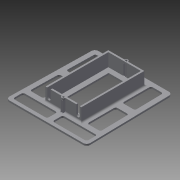
# Autodesk Inventor part: control pod layer b
Saved by Autodesk Inventor 2014 SP1 (Build 180222100, 222)
## iProperties
Created: 2017-06-28
Part Number: control pod layer b
Material: Generic
Document SubType Name: Modeling
Designer: kteo17
Density: 1 g/cm^3
Appearance: Default
Author: kteo17
Autodesk Inventor part; units mm, degrees
ref_plane "YZ Plane" through (0, 0, 0) normal (1, 0, 0) x (0, 1, 0)
ref_plane "XZ Plane" through (0, 0, 0) normal (0, 1, 0) x (-1, 0, 0)
ref_plane "XY Plane" through (0, 0, 0) normal (0, 0, 1) x (1, 0, 0)
sketch "Sketch1" plane through (0, 0, 0) normal (0, 0, 1) x (1, 0, 0)
  line L0 (3.175, 0) -> (146.685, 0)
  line L1 (149.86, 161.925) -> (0, 161.925)
  line L2 (0, 161.925) -> (3.175, 0)
  line L3 (149.86, 161.925) -> (146.685, 0)
  point P0 (0, 0)
  dimension "d74" = 161.925
  dimension "d75" = 143.51
  dimension "d76" = 149.86
  constraints: 8 end point, 1 horizontal, 1 parallel
  measures "d74" distance between parallel lines of L0 L1
  measures "d75" distance of L0.start L0.end
  measures "d76" distance of L1.start L1.end
extrude "Extrusion1" add sketch "Sketch1" along normal blind 3.048
fillet "Fillet1" radius 6.35 3 edges at (149.86, 161.925, 1.524) (146.685, 0, 1.524) (0, 161.925, 1.524)
sketch "Sketch4" plane through (0, 0, 3.048) normal (0, 0, 1) x (1, 0, 0)
  line L0 (44.7675, 16.764) -> (105.0925, 16.764)
  line L1 (105.0925, 16.764) -> (105.0925, 127)
  line L2 (105.0925, 127) -> (44.7675, 127)
  line L3 (44.7675, 127) -> (44.7675, 16.764)
  line L4 (44.7675, 16.764) -> (105.0925, 127) construction
  line L5 (105.0925, 16.764) -> (44.7675, 127) construction
  line L6 (41.5925, 13.589) -> (108.2675, 13.589)
  line L7 (108.2675, 13.589) -> (108.2675, 130.175)
  line L8 (108.2675, 130.175) -> (41.5925, 130.175)
  line L9 (41.5925, 130.175) -> (41.5925, 13.589)
  line L10 (193.675, 0) -> (193.675, 12.7)
  line L11 (3.175, 0) -> (140.4583, 0) projected
  point P0 (0, 0)
  dimension "d12" = 110.236
  dimension "d50" = 3.175
  dimension "d51" = 3.175
  dimension "d52" = 3.175
  dimension "d67" = 3.175
  dimension "d78" = 66.675
  dimension "d126" = 13.589
  constraints: 22 end point, 4 parallel, 2 horizontal, 2 perpendicular
  measures "d12" distance of L1.end L0.end
  measures "d50" distance between parallel lines of L2 L8
  measures "d51" distance between parallel lines of L7 L1
  measures "d52" distance between parallel lines of L0 L6
  measures "d67" distance between parallel lines of L9 L3
  measures "d78" distance of L7.end L8.end
  measures "d126" distance between parallel lines of L11 L6
extrude "Extrusion4" add sketch "Sketch4" along normal blind 24.13
sketch "Sketch5" plane through (0, 0, 27.178) normal (0, 0, 1) x (1, 0, 0)
  line L0 (41.5925, 13.589) -> (108.2675, 13.589) projected
  line L1 (108.2675, 130.175) -> (41.5925, 130.175) projected
  arc A0 (78.105, 130.175) -> (71.755, 130.175) centre (74.93, 130.175) ccw
  arc A1 (71.755, 13.589) -> (78.105, 13.589) centre (74.93, 13.589) ccw
  point P0 (0, 0)
  dimension "d127" = 3.175
  constraints: 4 point on circle, 4 point on line, 2 centre point, 2 midpoint
  measures "d127" radius of A0
extrude "Extrusion5" add sketch "Sketch5" against normal blind 3.175
sketch "Sketch6" plane through (41.5925, 130.175, 3.048) normal (0, 1, 0) x (1, 0, 0)
  line L0 (0, 0) -> (66.675, 0) projected
  line L1 (30.1625, -20.955) -> (36.5125, -20.955)
  line L2 (36.5125, -20.955) -> (36.5125, 0)
  line L3 (36.5125, 0) -> (30.1625, 0)
  line L4 (30.1625, 0) -> (30.1625, -20.955)
  point P0 (-41.5925, 3.048)
  constraints: 8 end point, 2 parallel, 1 horizontal, 1 perpendicular, 1 point on line
extrude "Extrusion6" cut sketch "Sketch6" against normal blind 127
sketch "Sketch9" plane through (0, 0, 27.178) normal (0, 0, 1) x (1, 0, 0)
  arc A0 (71.755, 13.589) -> (78.105, 13.589) centre (74.93, 13.589) ccw projected
  arc A1 (78.105, 130.175) -> (71.755, 130.175) centre (74.93, 130.175) ccw projected
  circle A2 centre (74.93, 130.175) radius 1.5875
  circle A3 centre (74.93, 13.589) radius 1.5875
  point P0 (0, 0)
  constraints: 2 centre point, 2 coincident
extrude "Extrusion9" cut sketch "Sketch9" against normal blind 2.54
sketch "Sketch10" plane through (108.2675, 130.175, 27.178) normal (0, 1, 0) x (1, 0, 0)
  line L0 (0, 0) -> (-30.1625, 0) projected
  line L1 (-3.175, 0) -> (-9.525, 0)
  line L2 (-9.525, 0) -> (-9.525, 15.875)
  line L3 (-6.35, 22.225) -> (-6.35, 22.225)
  line L4 (-3.175, 15.875) -> (-3.175, 0)
  line L5 (-63.5, 0) -> (-57.15, 0)
  line L6 (-57.15, 0) -> (-57.15, 15.875)
  line L7 (-60.325, 22.225) -> (-60.325, 22.225)
  line L8 (-63.5, 15.875) -> (-63.5, 0)
  arc A0 (-57.15, 15.875) -> (-63.5, 15.875) centre (-60.325, 15.875) ccw
  arc A1 (-3.175, 15.875) -> (-9.525, 15.875) centre (-6.35, 15.875) ccw
  point P0 (-108.2675, 27.178)
  constraints: 16 end point, 4 parallel, 4 point on circle, 2 centre point, 2 horizontal, 2 perpendicular, 2 point on line, 2 tangent
extrude "Extrusion10" cut sketch "Sketch10" against normal blind 25.4
fillet "Fillet3" radius 3.175 6 edges at (93.1863, 130.175, 3.048) (56.6738, 130.175, 3.048) (108.2675, 71.882, 3.048) (93.1863, 13.589, 3.048) (56.6738, 13.589, 3.048) (41.5925, 71.882, 3.048)
sketch "Sketch15" plane through (0, 0, 3.048) normal (0, 0, 1) x (1, 0, 0)
  line L0 (72.9998, 133.35) -> (74.0715, 133.35)
  line L1 (74.0715, 133.35) -> (74.0715, 126.111)
  line L2 (74.0715, 126.111) -> (72.9998, 126.111)
  line L3 (72.9998, 126.111) -> (72.9998, 133.35)
  line L4 (76.876, 133.35) -> (75.7704, 133.35)
  line L5 (75.7704, 133.35) -> (75.7704, 126.111)
  line L6 (75.7704, 126.111) -> (76.876, 126.111)
  line L7 (76.876, 126.111) -> (76.876, 133.35)
  line L8 (73.0082, 16.7637) -> (74.08, 16.7637)
  line L9 (74.08, 16.7637) -> (74.08, 10.4137)
  line L10 (74.08, 10.4137) -> (73.0082, 10.4137)
  line L11 (73.0082, 10.4137) -> (73.0082, 16.7637)
  line L12 (76.8845, 10.4137) -> (75.7789, 10.4137)
  line L13 (75.7789, 10.4137) -> (75.7789, 16.7637)
  line L14 (75.7789, 16.7637) -> (76.8845, 16.7637)
  line L15 (76.8845, 16.7637) -> (76.8845, 10.4137)
  point P0 (0, 0)
  constraints: 32 end point, 8 parallel, 4 horizontal, 4 perpendicular
extrude "Extrusion15" add sketch "Sketch15" along normal blind 20.7772
sketch "Sketch16" plane through (75.7704, 133.35, 3.048) normal (0, 1, 0) x (1, 0, 0)
  line L0 (-3.175, 0) -> (1.5875, 0)
  line L1 (1.5875, 0) -> (1.5875, -0.254)
  line L2 (1.5875, -0.254) -> (-3.175, -0.254)
  line L3 (-3.175, -0.254) -> (-3.175, 0)
  point P0 (-75.7704, 3.048)
  dimension "d58" = 0.254
  constraints: 8 end point, 2 parallel, 1 horizontal, 1 perpendicular
  measures "d58" distance of L0.end L1.end
extrude "Extrusion16" cut sketch "Sketch16" against normal blind 127
fillet "Fillet4" radius 6.35 1 edges at (3.175, 0, 1.524)
sketch "Sketch19" plane through (0, 0, 3.048) normal (0, 0, 1) x (1, 0, 0)
  line L0 (54.2925, 25.8383) -> (95.5675, 25.8383)
  line L1 (95.5675, 25.8383) -> (95.5675, 117.9257)
  line L2 (95.5675, 117.9257) -> (54.2925, 117.9257)
  line L3 (54.2925, 117.9257) -> (54.2925, 25.8383)
  line L4 (54.2925, 25.8383) -> (95.5675, 117.9257) construction
  line L5 (95.5675, 25.8383) -> (54.2925, 117.9257) construction
  point P0 (0, 0)
  point P1 (74.93, 71.882)
  constraints: 12 end point, 2 midpoint, 2 parallel, 1 horizontal, 1 perpendicular
extrude "Extrusion18" cut sketch "Sketch19" against normal blind 3.048
sketch "Sketch21" plane through (0, 0, 3.048) normal (0, 0, 1) x (1, 0, 0)
  arc A0 (149.733, 155.4505) -> (143.3843, 161.925) centre (143.3843, 155.575) ccw projected
  line L0 (143.3843, 139.7) -> (143.3843, 152.4)
  line L1 (6.4757, 152.4) -> (6.4757, 139.7)
  line L2 (79.8843, 152.4) -> (79.8843, 139.7)
  line L3 (69.9757, 152.4) -> (69.9757, 139.7)
  line L4 (140.2093, 155.575) -> (83.0593, 155.575)
  line L5 (66.8007, 155.575) -> (9.6507, 155.575)
  line L6 (9.6507, 136.525) -> (66.8007, 136.525)
  line L7 (83.0593, 136.525) -> (140.2093, 136.525)
  arc A1 (9.6507, 155.575) -> (6.4757, 152.4) centre (9.6507, 152.4) ccw
  arc A2 (6.4757, 139.7) -> (9.6507, 136.525) centre (9.6507, 139.7) ccw
  arc A3 (66.8007, 136.525) -> (69.9757, 139.7) centre (66.8007, 139.7) ccw
  arc A4 (69.9757, 152.4) -> (66.8007, 155.575) centre (66.8007, 152.4) ccw
  arc A5 (83.0593, 155.575) -> (79.8843, 152.4) centre (83.0593, 152.4) ccw
  arc A6 (79.8843, 139.7) -> (83.0593, 136.525) centre (83.0593, 139.7) ccw
  arc A7 (140.2093, 136.525) -> (143.3843, 139.7) centre (140.2093, 139.7) ccw
  arc A8 (143.3843, 152.4) -> (140.2093, 155.575) centre (140.2093, 152.4) ccw
  point P0 (0, 0)
  dimension "d97" = 3.175
  dimension "d111" = 19.05
  dimension "d112" = 19.05
  dimension "d113" = 63.5
  dimension "d114" = 63.5
  constraints: 16 end point, 16 point on circle, 16 tangent, 8 centre point, 7 equal radius, 6 perpendicular, 5 parallel, 2 horizontal, 2 point on line
  measures "d97" radius of A1
  measures "d111" distance between parallel lines of L6 L5
  measures "d112" distance between parallel lines of L4 L7
  measures "d113" distance between parallel lines of L3 L1
  measures "d114" distance between parallel lines of L0 L2
extrude "Extrusion20" cut sketch "Sketch21" against normal blind 3.048
sketch "Sketch22" plane through (0, 0, 3.048) normal (0, 0, 1) x (1, 0, 0)
  line L0 (66.8007, 136.525) -> (9.6507, 136.525) projected
  line L1 (146.8071, 6.2255) -> (149.733, 155.4505) projected
  line L2 (0.127, 155.4505) -> (3.0529, 6.2255) projected
  line L3 (31.115, 127) -> (12.6633, 127)
  line L4 (118.745, 127) -> (137.1967, 127)
  line L5 (15.5083, 7.9375) -> (31.75, 7.9375)
  line L6 (118.745, 7.9375) -> (134.9867, 7.9375)
  line L7 (13.5815, 73.8187) -> (31.115, 73.8187)
  line L8 (14.59, 61.1187) -> (31.75, 61.1187)
  line L9 (118.745, 61.1187) -> (135.905, 61.1187)
  line L10 (118.745, 73.8187) -> (136.2785, 73.8187)
  line L11 (9.4889, 123.7628) -> (10.4071, 76.9315)
  line L12 (11.4157, 57.8815) -> (12.3339, 11.0503)
  line L13 (34.29, 123.825) -> (34.29, 76.9937)
  line L14 (34.925, 57.9437) -> (34.925, 11.1125)
  line L15 (115.57, 123.825) -> (115.57, 76.9937)
  line L16 (115.57, 57.9437) -> (115.57, 11.1125)
  line L17 (140.3711, 123.7628) -> (139.4529, 76.9315)
  line L18 (139.0793, 57.8815) -> (138.1611, 11.0503)
  arc A0 (12.6633, 127) -> (9.4889, 123.7628) centre (12.6633, 123.825) ccw
  arc A1 (34.29, 123.825) -> (31.115, 127) centre (31.115, 123.825) ccw
  arc A2 (34.925, 57.9437) -> (31.75, 61.1187) centre (31.75, 57.9437) ccw
  arc A3 (14.59, 61.1187) -> (11.4157, 57.8815) centre (14.59, 57.9437) ccw
  arc A4 (12.3339, 11.0503) -> (15.5083, 7.9375) centre (15.5083, 11.1125) ccw
  arc A5 (31.75, 7.9375) -> (34.925, 11.1125) centre (31.75, 11.1125) ccw
  arc A6 (115.57, 11.1125) -> (118.745, 7.9375) centre (118.745, 11.1125) ccw
  arc A7 (134.9867, 7.9375) -> (138.1611, 11.0503) centre (134.9867, 11.1125) ccw
  arc A8 (139.0793, 57.8815) -> (135.905, 61.1187) centre (135.905, 57.9437) ccw
  arc A9 (118.745, 61.1187) -> (115.57, 57.9437) centre (118.745, 57.9437) ccw
  arc A10 (115.57, 76.9937) -> (118.745, 73.8187) centre (118.745, 76.9937) ccw
  arc A11 (136.2785, 73.8187) -> (139.4529, 76.9315) centre (136.2785, 76.9937) ccw
  arc A12 (140.3711, 123.7628) -> (137.1967, 127) centre (137.1967, 123.825) ccw
  arc A13 (118.745, 127) -> (115.57, 123.825) centre (118.745, 123.825) ccw
  arc A14 (31.115, 73.8187) -> (34.29, 76.9937) centre (31.115, 76.9937) ccw
  arc A15 (10.4071, 76.9315) -> (13.5815, 73.8187) centre (13.5815, 76.9937) ccw
  line L19 (38.4175, 133.35) -> (38.4175, 10.414) projected
  line L20 (111.4425, 10.414) -> (111.4425, 133.35) projected
  point P0 (0, 0)
  dimension "d107" = 3.175
  dimension "d108" = 3.175
  dimension "d122" = 4.1275
  dimension "d123" = 4.1275
  dimension "d124" = 4.1275
  constraints: 32 end point, 32 point on circle, 32 tangent, 16 centre point, 14 equal radius, 10 perpendicular, 8 parallel, 2 collinear
  measures "d107" radius of A0
  measures "d108" radius of A14
  measures "d122" distance between parallel lines of L19 L13
  measures "d123" distance between parallel lines of L20 L15
  measures "d124" distance between parallel lines of L20 L16
extrude "Extrusion21" cut sketch "Sketch22" against normal blind 3.048
body "Solid1"
